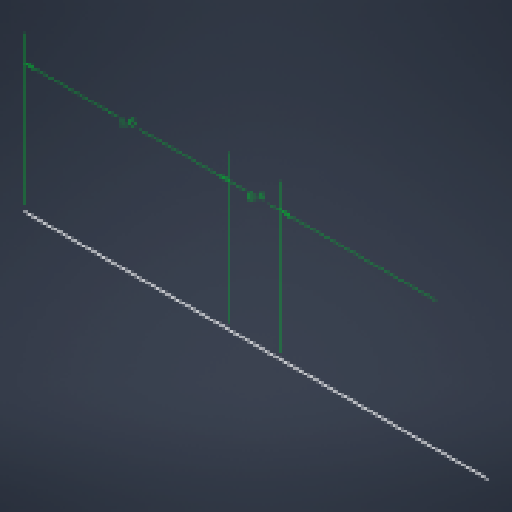
# Autodesk Inventor part: Part6
Saved by Autodesk Inventor 2026 (Build 300175000, 175)
## iProperties
Created: 2025-10-10
Part Number: Part6
Material: Generic
Document SubType Name: Modeling
Designer: kenny
Density: 1 g/cm^3
Appearance: Default
Author: kenny
Autodesk Inventor part; units mm, degrees
ref_plane "YZ Plane" through (0, 0, 0) normal (1, 0, 0) x (0, 1, 0)
ref_plane "XZ Plane" through (0, 0, 0) normal (0, 1, 0) x (-1, 0, 0)
ref_plane "XY Plane" through (0, 0, 0) normal (0, 0, 1) x (1, 0, 0)
sketch "Sketch1" plane through (0, 0, 0) normal (0, 0, 1) x (1, 0, 0)
  line L0 (0, 0) -> (-1.6043, 0)
  line L1 (-1.6043, 0) -> (-2.0043, 0)
  line L2 (-2.0043, 0) -> (-3.6043, 0)
  line L3 (0, 0) -> (0, -15)
  line L4 (0, -15) -> (-3.6043, -15)
  line L5 (-3.6043, -15) -> (-3.6043, 0)
  line L6 (0, 0) -> (0, 18.6)
  line L7 (0, 18.6) -> (-3.6043, 18.6)
  line L8 (-3.6043, 18.6) -> (-3.6043, 0)
  line L9 (-2.0043, 0) -> (-2.0043, -15)
  line L10 (-2.0043, 0.2824) -> (-2.0043, 18.6)
  line L11 (0, -15) -> (49.6, -15)
  line L12 (49.6, -15) -> (50, -15)
  line L13 (50, -15) -> (51.6, -15)
  line L14 (51.6, -15) -> (51.6, 18.6)
  line L15 (51.6, 18.6) -> (50, 18.6)
  line L16 (50, 18.6) -> (50, -15)
  line L17 (50, 18.6) -> (-2.0043, 18.6)
  dimension "d0" = 0.4
  dimension "d1" = 1.6
  dimension "d2" = 15
  dimension "d4" = 49.6
  dimension "d5" = 0.4
  dimension "d6" = 1.6
  constraints: 36 end point, 8 perpendicular, 8 point on line, 2 horizontal, 2 vertical, 1 collinear
  measures "d0" distance of L0.end L1.end
  measures "d1" distance of L1.end L2.end
  measures "d2" distance of L0.start L3.end
  measures "d4" distance of L3.end L11.end
  measures "d5" distance of L11.end L12.end
  measures "d6" distance of L12.end L13.end
extrude "Extrusion1" add sketch "Sketch1" along normal blind 1.6
sketch "Sketch2" plane through (0, 0, 0) normal (0, 0, -1) x (-1, 0, 0)
  line L0 (3.6043, 18.6) -> (3.6043, -15) projected
  line L1 (3.6043, 18.6) -> (2.0043, 18.6)
  line L2 (-51.6, 18.6) -> (3.6043, 18.6) projected
  line L3 (2.0043, 18.6) -> (2.0043, -15)
  line L4 (3.6043, -15) -> (-51.6, -15) projected
  line L5 (-51.6, -15) -> (-51.6, 18.6) projected
  line L6 (-51.6, 18.6) -> (-50, 18.6)
  line L7 (-50, 18.6) -> (-50, -15)
  line L8 (-51.6, 18.6) -> (-50, 18.6)
  line L9 (-51.6, -15) -> (-50, -15)
  line L10 (2.0043, 18.6) -> (3.6043, 18.6)
  line L11 (3.6043, -15) -> (2.0043, -15)
  point P0 (0, 0)
  dimension "d9" = 1.6
  dimension "d10" = 1.6
  constraints: 16 end point, 5 equal length, 3 point on line, 1 perpendicular
  measures "d9" distance of L0.start L1.end
  measures "d10" distance of L2.start L6.end
extrude "Extrusion2" add sketch "Sketch2" along normal blind 14.6 contours L0 L4 L3 L1 | L7 L4 L5 L2
sketch "Sketch3" plane through (-3.6043, -15, 1.6) normal (-1, 0, 0) x (0, 0, 1)
  line L0 (-16.2, 0) -> (0, 0) projected
  line L1 (0, 0) -> (0, 5)
  line L2 (0, 33.6) -> (0, 0) projected
  line L3 (0, 0) -> (-6.6, 0)
  line L4 (-1.6, 0) -> (-16.2, 0) projected
  line L5 (-6.6, 0) -> (-6.6, 5)
  circle A0 centre (-6.6, 5) radius 2.15
  point P0 (-1.6, 15)
  dimension "d13" = 5
  dimension "d14" = 6.6
  dimension "d15" = 4.3
  constraints: 6 end point, 2 point on line, 1 centre point, 1 coincident, 1 vertical
  measures "d13" distance of L0.end L1.end
  measures "d14" distance of L0.end L3.end
  measures "d15" diameter of A0
extrude "Extrusion3" cut sketch "Sketch3" against normal blind 68.6
sketch "Sketch4" plane through (0, 0, 1.6) normal (0, 0, 1) x (1, 0, 0)
  line L0 (19.036, -6.8706) -> (33.9718, -6.8706)
  line L1 (33.9718, -6.8706) -> (33.9718, -8.566)
  line L2 (33.9718, -8.566) -> (19.036, -8.566)
  line L3 (19.036, -8.566) -> (19.036, -6.8706)
  point P0 (0, 0)
  constraints: 8 end point, 2 parallel, 1 horizontal, 1 perpendicular
extrude "Extrusion4" cut sketch "Sketch4" against normal blind 68.6
body "Solid1"
